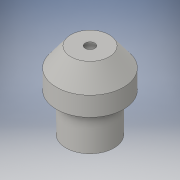
# Autodesk Inventor part: Nozzle
Saved by Autodesk Inventor 2016 (Build 200138000, 138)
## iProperties
Created: 2015-07-08
Part Number: Nozzle
Material: Generic
Document SubType Name: Modeling
Designer: Scott
Density: 1 g/cm^3
Appearance: Default
Author: Scott
Autodesk Inventor part; units mm, degrees
ref_plane "YZ Plane" through (0, 0, 0) normal (1, 0, 0) x (0, 1, 0)
ref_plane "XZ Plane" through (0, 0, 0) normal (0, 1, 0) x (-1, 0, 0)
ref_plane "XY Plane" through (0, 0, 0) normal (0, 0, 1) x (1, 0, 0)
sketch "Sketch1" plane through (0, 0, 0) normal (0, 1, 0) x (-1, 0, 0)
  circle A0 centre (0, 0) radius 3.175
  circle A1 centre (0, 0) radius 1.905
  dimension "d0" = 6.35
  dimension "d1" = 3.81
  constraints: 2 centre point, 2 coincident
  measures "d0" diameter of A0
  measures "d1" diameter of A1
extrude "Extrusion1" add sketch "Sketch1" along normal blind 7.62
sketch "Sketch2" plane through (0, 7.62, 0) normal (0, 1, 0) x (1, 0, 0)
  point P0 (0, 0)
sketch "Sketch3" plane through (0, 0, 0) normal (0, 0, 1) x (1, 0, 0)
  line L0 (3.175, 7.62) -> (-3.175, 7.62) projected
  line L1 (0, 7.62) -> (0, 10.16)
  line L2 (0, 10.16) -> (0.635, 10.16)
  line L3 (4.445, 7.62) -> (2.54, 10.16)
  line L4 (2.54, 10.16) -> (0.635, 10.16)
  line L5 (4.445, 7.62) -> (4.445, 5.08)
  line L6 (4.445, 5.08) -> (3.175, 5.08)
  line L7 (3.175, 0) -> (3.175, 7.62) projected
  line L8 (3.175, 7.62) -> (3.175, 5.08)
  line L9 (0.635, 10.16) -> (1.905, 7.62)
  line L10 (3.175, 7.62) -> (1.905, 7.62)
  point P0 (0, 0)
  dimension "d4" = 2.54
  dimension "d5" = 0.635
  dimension "d6" = 1.27
  constraints: 18 end point, 3 collinear, 3 point on line, 2 perpendicular, 2 vertical, 1 midpoint
  measures "d4" distance of L1.start L1.end
  measures "d5" distance of L1.end L2.end
  measures "d6" distance of L0.start L3.start
revolve "Revolution1" add sketch "Sketch3" angle 360 about axis through (0, 7.62, 0) along (0, 1, 0) contours L0 L9 L4 L3 L5 L6 L7
body "Solid1"
